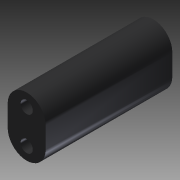
# Autodesk Inventor part: Front mount
Saved by Autodesk Inventor 2015 (Build 190159000, 159)
## iProperties
Created: 2016-10-31
Part Number: Front mount
Material: ABS Plastic
Document SubType Name: Modeling
Designer: James Yelland
Density: 1.06 g/cm^3
Appearance: Smooth - White
Mass: 7.98828 g
Surface Area: 62.2612 cm^2
Volume: 7.53611 cm^3
Author: James Yelland
Autodesk Inventor part; units mm, degrees
ref_plane "YZ Plane" through (0, 0, 0) normal (1, 0, 0) x (0, 1, 0)
ref_plane "XZ Plane" through (0, 0, 0) normal (0, 1, 0) x (-1, 0, 0)
ref_plane "XY Plane" through (0, 0, 0) normal (0, 0, 1) x (1, 0, 0)
sketch "Sketch2" plane through (0, 0, 0) normal (0, 1, 0) x (-1, 0, 0)
  line L0 (-4.5, -10) -> (-4.5, -5)
  line L1 (4.5, -10) -> (4.5, -5)
  arc A0 (4.5, -5) -> (-4.5, -5) centre (0, -5) ccw
  arc A1 (-4.5, -10) -> (4.5, -10) centre (0, -10) ccw
  point P0 (0, 0)
  point P1 (0.9888, -13.1808)
  dimension "d75" = 5
  dimension "d76" = 5
  constraints: 4 end point, 4 point on circle, 2 centre point, 1 vertical
  measures "d75" distance of L0.start L0.end
  measures "d76" distance of L1.start L1.end
extrude "Extrusion1" add sketch "Sketch2" along normal blind 30
sketch "Sketch14" plane through (-4.5, 0, -10) normal (-1, 0, 0) x (0, 0, 1)
  line L0 (-4.5, 0) -> (-4.5, 30) projected
  line L1 (-4.5, 0) -> (-4.5, 15)
  line L2 (-4.5, 15) -> (2, 15)
  circle A0 centre (2, 15) radius 2.25
  point P0 (10, 0)
  point P1 (-11.5, 30)
  dimension "d80" = 15
  dimension "d81" = 6.5
  dimension "d82" = 4.5
  constraints: 4 end point, 1 centre point, 1 coincident, 1 midpoint, 1 perpendicular
  measures "d80" distance of L0.start L1.end
  measures "d81" distance of L1.end L2.end
  measures "d82" diameter of A0
extrude "Extrusion13" cut sketch "Sketch14" against normal blind 5
sketch "Sketch18" plane through (0, 30, 0) normal (0, 1, 0) x (1, 0, 0)
  arc A0 (4.5, 10) -> (-4.5, 10) centre (0, 10) ccw projected
  line L0 (0, 14.5) -> (0, 11.5)
  circle A1 centre (0, 11.5) radius 1.45
  arc A2 (-4.5, 5) -> (4.5, 5) centre (0, 5) ccw projected
  line L1 (0, 0.5) -> (0, 3.5)
  circle A3 centre (0, 3.5) radius 1.45
  point P0 (0, 0)
  dimension "d103" = 3
  dimension "d104" = 2.9
  dimension "d105" = 3
  dimension "d106" = 2.9
  constraints: 4 end point, 2 centre point, 2 coincident, 2 point on circle, 2 vertical
  measures "d103" distance of L0.start L0.end
  measures "d104" diameter of A1
  measures "d105" distance of L1.start L1.end
  measures "d106" diameter of A3
extrude "Extrusion17" cut sketch "Sketch18" against normal blind 10
sketch "Sketch19" plane through (0, 0, 0) normal (0, -1, 0) x (1, 0, 0)
  line L0 (4.5, -10) -> (4.5, -5) projected
  arc A0 (4.5, -5) -> (-4.5, -5) centre (0, -5) ccw projected
  line L1 (-4.5, -5) -> (-4.5, -10) projected
  arc A1 (-4.5, -10) -> (4.5, -10) centre (0, -10) ccw projected
  circle A2 centre (0, -11.5) radius 1.45 projected
  circle A3 centre (0, -3.5) radius 1.45 projected
extrude "Extrusion18" cut sketch "Sketch19" against normal blind 10 contours A2 | A3
body "Solid1"
